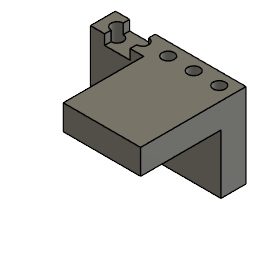
DisplaySupport (Autodesk Fusion 360 design; units mm, degrees)
Autodesk Fusion 360 part; units mm, degrees
sketch "Skizze1" plane through (0, 0, 0) normal (0, 1, 0) x (1, 0, 0)
  circle A0 centre (0, 0) radius 0.6
  circle A1 centre (2.54, 0) radius 0.6
  circle A2 centre (5.08, 0) radius 0.6
  circle A3 centre (7.62, 0) radius 0.6
  circle A4 centre (10.16, 0) radius 0.6
  line L0 (11.58, 1.25) -> (-1.42, 1.25)
  line L1 (-1.42, 1.25) -> (-1.42, -1.25)
  line L2 (-1.42, -1.25) -> (11.58, -1.25)
  line L3 (11.58, -1.25) -> (11.58, 1.25)
  line L4 (11.58, 1.25) -> (-1.42, -1.25) construction
  line L5 (-1.42, 1.25) -> (11.58, -1.25) construction
  point P0 (5.08, 0)
  dimension "d1" = 1.2
  dimension "d4" = 2.54
  dimension "d5" = 0
  dimension "d6" = 13
  dimension "d7" = 2.5
  constraint coincident A0.centre origin
  constraint horizontal L0
  constraint perpendicular L0 L1
  constraint parallel L0 L2
  constraint parallel L1 L3
  constraint coincident L4 P0
  constraint coincident L5 P0
  constraint coincident P0 A2.centre
  measures "d1" diameter of A0
  measures "d6" distance of L1.end L2.end
  measures "d7" distance of L0.end L1.end
extrude "Extrusion1" add sketch "Skizze1" along normal blind 8.4
sketch "Skizze4" plane through (0, 0, 1.25) normal (0, 0, 1) x (1, 0, 0)
  line L0 (-1.42, 0) -> (11.58, 0)
  line L1 (11.58, 0) -> (11.58, 8.4)
  line L2 (11.58, 8.4) -> (-1.42, 8.4)
  line L3 (-1.42, 8.4) -> (-1.42, 0)
  line L4 (11.58, 8.4) -> (3.88, 8.4)
  line L5 (3.88, 8.4) -> (3.88, 5.9)
  line L6 (3.88, 5.9) -> (11.58, 5.9)
  line L7 (11.58, 5.9) -> (11.58, 8.4)
  dimension "d10" = 7.7
  dimension "d11" = 2.5
  constraint horizontal L4
  constraint vertical L5
  constraint horizontal L6
  constraint vertical L7
  constraint coincident L1.end L2.start
  measures "d10" distance of L1.end L4.end
  measures "d11" distance of L1.end L6.end
extrude "Extrusion2" add sketch "Skizze4" along normal blind 8 contours L1 L2 L4 L5 L6 L7
sketch "Skizze5" plane through (0, 8.4, 0) normal (0, 1, 0) x (-1, 0, 0)
  circle A0 centre (-7.62, 0) radius 0.6
  circle A1 centre (-5.08, 0) radius 0.6
  circle A2 centre (-10.16, 0) radius 0.6
  circle A3 centre (-2.54, 0) radius 0.6
  circle A4 centre (0, 0) radius 0.6
  line L0 (-11.58, 9.25) -> (-11.58, -1.25)
  line L1 (-11.58, -1.25) -> (1.42, -1.25)
  line L2 (1.42, -1.25) -> (1.42, 1.25)
  line L3 (1.42, 1.25) -> (-3.88, 1.25)
  line L4 (-3.88, 1.25) -> (-3.88, 9.25)
  line L5 (-3.88, 9.25) -> (-11.58, 9.25)
  line L6 (0, -1.25) -> (-2.54, -1.25)
  line L7 (-2.54, -1.25) -> (-2.54, 1.25)
  line L8 (-2.54, 1.25) -> (0, 1.25)
  line L9 (0, 1.25) -> (0, -1.25)
  constraint horizontal L6
  constraint vertical L7
  constraint horizontal L8
  constraint vertical L9
  constraint coincident L3 L7.end
  constraint coincident L1 L6.start
extrude "Extrusion3" cut sketch "Skizze5" against normal blind 1 contours A3 A4 L1 L3 L6 L7 L8 L9
